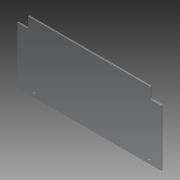
# Autodesk Inventor part: GE-13042
Saved by Autodesk Inventor 2013 (Build 170138000, 138)
## iProperties
Created: 2013-01-06
Part Number: GE-13042
Material: Polycarbonate, Clear
Document SubType Name: Modeling
Designer: Phillip
Density: 1 g/cm^3
Author: Phillip
Autodesk Inventor part; units mm, degrees
ref_plane "YZ Plane" through (0, 0, 0) normal (1, 0, 0) x (0, 1, 0)
ref_plane "XZ Plane" through (0, 0, 0) normal (0, 1, 0) x (-1, 0, 0)
sketch "Sketch1" plane through (0, 0, 0) normal (0, 0, 1) x (1, 0, 0)
  line L0 (-295.275, -138.176) -> (295.275, -138.176)
  line L1 (295.275, -138.176) -> (295.275, 138.176)
  line L2 (295.275, 138.176) -> (-295.275, 138.176)
  line L3 (-295.275, 138.176) -> (-295.275, -138.176)
  line L4 (-295.275, -138.176) -> (295.275, 138.176) construction
  line L5 (295.275, -138.176) -> (-295.275, 138.176) construction
  point P0 (0, 0)
  dimension "d0" = 590.55
  dimension "d1" = 276.352
  constraints: 12 end point, 2 midpoint, 2 parallel, 1 horizontal, 1 perpendicular
  measures "d0" distance of L2.end L1.end
  measures "d1" distance of L1.end L0.end
extrude "Extrusion1" add sketch "Sketch1" against normal blind 6.35
sketch "Sketch2" plane through (0, 0, 0) normal (0, 0, 1) x (1, 0, 0)
  line L0 (-295.275, -138.176) -> (295.275, -138.176) projected
  line L1 (295.275, 138.176) -> (-295.275, 138.176) projected
  line L2 (-295.275, 138.176) -> (-295.275, -138.176) projected
  line L3 (-295.275, 93.726) -> (-250.825, 93.726)
  line L4 (-250.825, 93.726) -> (-250.825, 138.176)
  point P0 (0, 0)
  dimension "d4" = 44.45
  dimension "d6" = 231.902
  constraints: 4 end point, 2 perpendicular, 2 point on line
  measures "d4" distance of L3.start L3.end
  measures "d6" distance between parallel lines of L3 L0
extrude "Extrusion2" cut sketch "Sketch2" against normal through all
fillet "Fillet1" radius 6.35 1 edges at (-250.825, 93.726, -3.175)
ref_plane "Work Plane1" through (0, -138.176, 0) normal (1, 0, 0) x (0, 1, 0)
mirror "Mirror1" about plane through (0, -138.176, 0) normal (1, 0, 0) of "Extrusion2", "Fillet1"
sketch "Sketch3" plane through (0, 0, 0) normal (0, 0, 1) x (1, 0, 0)
  line L0 (-295.275, 93.726) -> (-295.275, -138.176) projected
  line L1 (-295.275, -138.176) -> (295.275, -138.176) projected
  point P0 (0, 0)
  point P1 (-228.473, -122.174)
  point P2 (244.475, -122.174)
  dimension "d10" = 66.802
  dimension "d11" = 539.75
  dimension "d12" = 16.002
  constraints: 1 horizontal alignment
  measures "d10" distance from line of point (-228.473, -122.174) L0
  measures "d11" distance from line of point (244.475, -122.174) L0
  measures "d12" distance from line of point (-228.473, -122.174) L1
hole "Hole1" at (-228.473, -122.174, 0) at (244.475, -122.174, 0) direction (0, 0, -1) diameter 6.858 end through all
body "Solid1"
